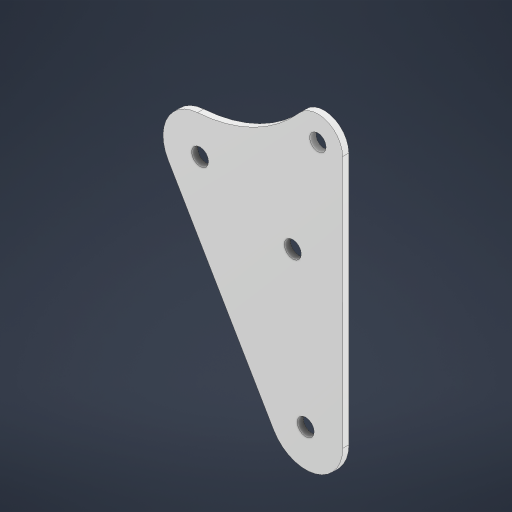
# Autodesk Inventor part: pod_gusset
Saved by Autodesk Inventor 2024 (Build 280153000, 153)
## iProperties
Created: 2024-01-18
Part Number: pod_gusset
Material: Acetal Resin, White
Document SubType Name: Modeling
Designer: avere
Density: 1.425 g/cm^3
Appearance: Smooth - White
Author: avere
Autodesk Inventor part; units mm, degrees
ref_plane "YZ Plane" through (0, 0, 0) normal (1, 0, 0) x (0, 1, 0)
ref_plane "XZ Plane" through (0, 0, 0) normal (0, 1, 0) x (-1, 0, 0)
ref_plane "XY Plane" through (0, 0, 0) normal (0, 0, 1) x (1, 0, 0)
sketch "main" plane through (0, 0, 0) normal (0, 0, 1) x (1, 0, 0)
  line L0 (-30.6986, 36.9894) -> (-3.5098, -9.6529)
  line L1 (14.2033, 60.1599) -> (14.2442, -4.8501)
  circle A0 centre (4.7192, -4.8561) radius 2.1844
  arc A1 (-3.5098, -9.6529) -> (14.2442, -4.8501) centre (4.7192, -4.8561) ccw
  line L2 (4.7192, -4.8561) -> (42.8192, -4.8561) construction
  circle A2 centre (1.3985, 33.099) radius 2.1844
  line L3 (4.7192, -4.8561) -> (69.8067, -4.8561) construction
  circle A3 centre (7.8533, 60.1559) radius 2.1209
  arc A4 (14.2033, 60.1599) -> (3.0678, 64.3299) centre (7.8533, 60.1559) ccw
  line L4 (1.3985, 33.099) -> (26.7985, 33.099) construction
  circle A5 centre (-22.4696, 41.7863) radius 2.1844
  arc A6 (-23.1365, 51.2879) -> (-30.6986, 36.9894) centre (-22.4696, 41.7863) ccw
  arc A7 (-23.1365, 51.2879) -> (3.0678, 64.3299) centre (-25.8203, 89.5265) ccw
  point P0 (-13.3913, 7.903)
  dimension "d33" = 19.05
  dimension "d41" = 4.3688
  dimension "d48" = 12.7
  dimension "d52" = 19.05
  measures "d33" diameter of A1
  measures "d41" diameter of A2
  measures "d48" diameter of A4
  measures "d52" diameter of A6
sketch "Sketch1" plane through (0, 0, 0) normal (0, 0, 1) x (1, 0, 0)
  line L0 (-25.5568, 5.0437) -> (1.632, -41.5986)
  line L1 (19.3451, 28.2142) -> (19.386, -36.7958)
  circle A0 centre (9.861, -36.8018) radius 2.1844
  arc A1 (1.632, -41.5986) -> (19.386, -36.7958) centre (9.861, -36.8018) ccw
  line L2 (9.861, -36.8018) -> (47.961, -36.8018) construction
  circle A2 centre (6.5404, 1.1532) radius 2.1844
  line L3 (9.861, -36.8018) -> (74.9485, -36.8018) construction
  circle A3 centre (12.9951, 28.2102) radius 2.1209
  arc A4 (19.3451, 28.2142) -> (8.2097, 32.3842) centre (12.9951, 28.2102) ccw
  line L4 (6.5404, 1.1532) -> (31.9404, 1.1532) construction
  circle A5 centre (-17.3278, 9.8406) radius 2.1844
  arc A6 (-17.9947, 19.3422) -> (-25.5568, 5.0437) centre (-17.3278, 9.8406) ccw
  arc A7 (-17.9947, 19.3422) -> (8.2097, 32.3842) centre (-20.6785, 57.5808) ccw
  point P0 (0, 0)
extrude "Extrusion1" add sketch "Sketch1" along normal blind 1.5875
body "Solid1"
